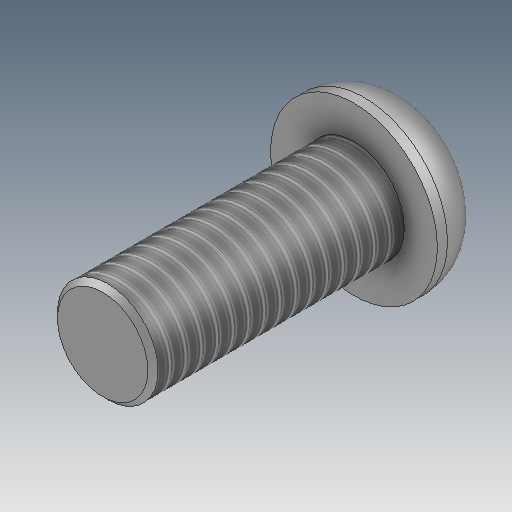
# Autodesk Inventor part: Tornillo allen cabeza boton M8x20mm
Saved by Autodesk Inventor 2020 (Build 240168000, 168)
## iProperties
Created: 2020-05-15
Part Number: Tornillo allen cabeza boton M8x20mm
Material: Generic
Document SubType Name: Modeling
Designer: Dante
Density: 1 g/cm^3
Appearance: Goma - Negro - Versión 1.1
Mass: 3.07248 g
Surface Area: 15.975 cm^2
Volume: 3.07248 cm^3
Author: Dante
Autodesk Inventor part; units mm, degrees
ref_plane "YZ Plane" through (0, 0, 0) normal (1, 0, 0) x (0, 1, 0)
ref_plane "XZ Plane" through (0, 0, 0) normal (0, 1, 0) x (-1, 0, 0)
ref_plane "XY Plane" through (0, 0, 0) normal (0, 0, 1) x (1, 0, 0)
sketch "Sketch1" plane through (0, 0, 0) normal (0, 0, 1) x (1, 0, 0)
  circle A0 centre (0, 0) radius 6.635
  circle A1 centre (0, 0) radius 4
  dimension "d0" = 13.27
  dimension "d1" = 8
  constraints: 2 centre point, 2 coincident
  measures "d0" diameter of A0
  measures "d1" diameter of A1
extrude "Extrusion1" add sketch "Sketch1" along normal blind 4.4
extrude "Extrusion2" add sketch "Sketch1" along normal blind 24.4 contours A1
sketch "Boceto2" plane through (0, 0, 0) normal (0, 0, -1) x (-1, 0, 0)
  line L0 (2.2909, 1.7564) -> (2.6666, -1.1058)
  line L1 (2.6666, -1.1058) -> (0.3756, -2.8622)
  line L2 (0.3756, -2.8622) -> (-2.2909, -1.7564)
  line L3 (-2.2909, -1.7564) -> (-2.6666, 1.1058)
  line L4 (-2.6666, 1.1058) -> (-0.3756, 2.8622)
  line L5 (-0.3756, 2.8622) -> (2.2909, 1.7564)
  point P0 (0, 0)
  point P1 (0, 0)
  dimension "d6" = 5
  constraints: 12 end point, 1 coincident, 13 other
  measures "d6" distance between parallel lines of L1 L4
extrude "Extrusión3" cut sketch "Boceto2" against normal blind 2.6
thread "Rosca1" size "M8x1.25" class "6g" standard "ISO Metric profile" length 430
fillet "Empalme1" radius 3.6 1 edges at (-6.635, 0, 0)
chamfer "Chaflán2" distance 0.4 angle 45 1 edges at (-4, 0, 24.4)
body "Solid1"
